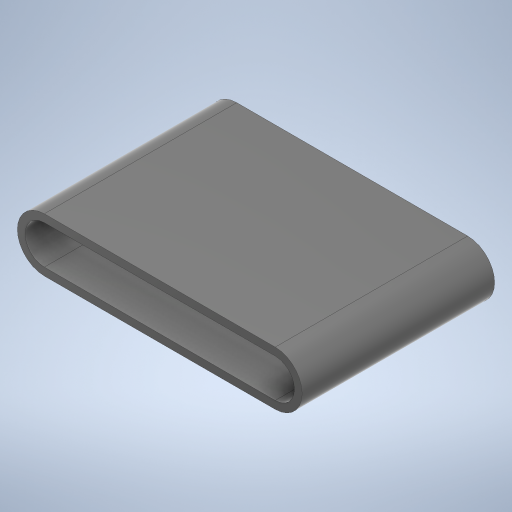
# Autodesk Inventor part: banda 1
Saved by Autodesk Inventor 2023 (Build 270158000, 158)
## iProperties
Created: 2022-04-05
Part Number: banda 1
Material: Genérico
Document SubType Name: Modeling
Designer: isaac
Density: 1 g/cm^3
Appearance: Valor por defecto
Author: isaac
Autodesk Inventor part; units mm, degrees
ref_plane "YZ Plane" through (0, 0, 0) normal (1, 0, 0) x (0, 1, 0)
ref_plane "XZ Plane" through (0, 0, 0) normal (0, 1, 0) x (-1, 0, 0)
ref_plane "XY Plane" through (0, 0, 0) normal (0, 0, 1) x (1, 0, 0)
sketch "Boceto1" plane through (0, 0, 0) normal (0, 0, 1) x (1, 0, 0)
  arc A0 (-300, 50) -> (-300, -50) centre (-300, 0) ccw
  arc A1 (300, -50) -> (300, 50) centre (300, 0) ccw
  line L0 (300, 50) -> (-300, 50)
  line L1 (-300, -50) -> (300, -50)
  line L2 (-300, 70) -> (300, 70)
  arc A2 (300, -70) -> (300, 70) centre (300, 0) ccw
  line L3 (300, -70) -> (-300, -70)
  arc A3 (-300, 70) -> (-300, -70) centre (-300, 0) ccw
  point P0 (0, 0)
  dimension "d0" = 300
  dimension "d1" = 300
  dimension "d2" = 100
  dimension "d3" = 100
  dimension "d4" = 20
  dimension "d5" = 20
  constraints: 8 end point, 8 point on circle, 6 tangent, 4 centre point, 2 horizontal, 2 horizontal alignment, 2 parallel, 1 concentric
  measures "d0" distance of point (0, 0) A0.centre
  measures "d1" distance of point (0, 0) A1.centre
  measures "d2" diameter of A0
  measures "d3" diameter of A1
  measures "d4" distance between parallel lines of L0 L2
  measures "d5" radial gap between concentric circles of A0 A3
extrude "Extrusión1" add sketch "Boceto1" along normal blind 500
